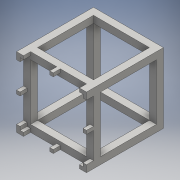
# Autodesk Inventor part: Kens_cube_of_fun_design_withpegs_spencermical
Saved by Autodesk Inventor 2016 (Build 200138000, 138)
## iProperties
Created: 2016-02-27
Part Number: Kens_cube_of_fun_design_withpegs_spencermical
Material: Generic
Document SubType Name: Modeling
Designer: Spencer
Density: 1 g/cm^3
Appearance: Default
Author: Spencer
Autodesk Inventor part; units mm, degrees
ref_plane "YZ Plane" through (0, 0, 0) normal (1, 0, 0) x (0, 1, 0)
ref_plane "XZ Plane" through (0, 0, 0) normal (0, 1, 0) x (-1, 0, 0)
ref_plane "XY Plane" through (0, 0, 0) normal (0, 0, 1) x (1, 0, 0)
sketch "Sketch1" plane through (0, 0, 0) normal (0, 1, 0) x (-1, 0, 0)
  line L0 (50, -50) -> (-50, -50)
  line L1 (-50, -50) -> (-50, 50)
  line L2 (-50, 50) -> (50, 50)
  line L3 (50, 50) -> (50, -50)
  point P0 (0, 0)
  dimension "d0" = 100
  dimension "d1" = 100
  dimension "d2" = 50
  dimension "d3" = 50
  constraints: 8 end point, 2 parallel, 1 horizontal, 1 perpendicular
  measures "d0" distance of L0.start L0.end
  measures "d1" distance of L2.end L0.start
  measures "d2" horizontal distance of L0.end point (0, 0)
  measures "d3" distance from line of L2 point (0, 0)
extrude "Extrusion1" add sketch "Sketch1" along normal blind 100
sketch "Sketch2" plane through (-50, 0, 50) normal (0, 0, 1) x (1, 0, 0)
  line L0 (10, 90) -> (90, 90)
  line L1 (90, 90) -> (90, 10)
  line L2 (90, 10) -> (10, 10)
  line L3 (10, 10) -> (10, 90)
  line L4 (100, 0) -> (0, 0) projected
  line L5 (100, 0) -> (100, 100) projected
  point P0 (50, 0)
  dimension "d6" = 80
  dimension "d7" = 10
  dimension "d8" = 80
  dimension "d9" = 10
  constraints: 8 end point, 2 parallel, 1 horizontal, 1 perpendicular
  measures "d6" distance of L2.end L0.start
  measures "d7" distance from line of L4 L2.end
  measures "d8" distance of L1.end L2.end
  measures "d9" distance from line of L5 L1.end
extrude "Extrusion2" cut sketch "Sketch2" against normal blind 100
sketch "Sketch3" plane through (50, 0, 50) normal (1, 0, 0) x (0, 0, -1)
  line L0 (10, 90) -> (90, 90)
  line L1 (90, 90) -> (90, 10)
  line L2 (90, 10) -> (10, 10)
  line L3 (10, 10) -> (10, 90)
  line L4 (0, 100) -> (100, 100) projected
  line L5 (100, 0) -> (100, 100) projected
  point P0 (50, 0)
  dimension "d12" = 80
  dimension "d13" = 10
  dimension "d14" = 80
  dimension "d15" = 10
  constraints: 8 end point, 2 parallel, 1 horizontal, 1 perpendicular
  measures "d12" distance of L2.end L0.start
  measures "d13" distance from line of L4 L0.start
  measures "d14" distance of L0.start L0.end
  measures "d15" distance from line of L5 L1.end
extrude "Extrusion3" cut sketch "Sketch3" against normal blind 100
sketch "Sketch4" plane through (0, 100, 0) normal (0, 1, 0) x (1, 0, 0)
  line L0 (-40, -50) -> (-40, -40) projected
  line L1 (50, 40) -> (40, 40) projected
  line L2 (-40, -40) -> (40, -40)
  line L3 (40, -40) -> (40, 40)
  line L4 (40, 40) -> (-40, 40)
  line L5 (-40, 40) -> (-40, -40)
  point P0 (0, 0)
  constraints: 8 end point, 2 parallel, 1 horizontal, 1 perpendicular
extrude "Extrusion4" cut sketch "Sketch4" against normal blind 100
sketch "Sketch9" plane through (0, 0, 0) normal (0, -1, 0) x (1, 0, 0)
  line L0 (50, 0.0049) -> (45, 0.0049)
  line L1 (45, 0.0049) -> (45, -2.4951)
  line L2 (45, -2.4951) -> (50, -2.4951)
  line L3 (50, -2.4951) -> (50, 0.0049)
  line L4 (40, 40) -> (40, -40) projected
  point P0 (0, 0)
  dimension "d40" = 5
  dimension "d41" = 5
  dimension "d42" = 2.5
  constraints: 8 end point, 2 parallel, 1 horizontal, 1 perpendicular
  measures "d40" distance from line of L4 L1.end
  measures "d41" distance of L1.end L2.end
  measures "d42" distance of L0.end L1.end
sketch "Sketch10" plane through (0, 0, 0) normal (0, -1, 0) x (1, 0, 0)
  line L0 (50, -40) -> (50, 40) projected
  line L1 (50, 0) -> (45, 0)
  line L2 (45, 0) -> (45, 2.5)
  line L3 (45, 2.5) -> (50, 2.5)
  line L4 (50, 2.5) -> (50, 0)
  line L5 (40, 40) -> (40, -40) projected
  point P0 (0, 0)
  dimension "d43" = 2.5
  dimension "d44" = 5
  constraints: 8 end point, 2 parallel, 1 horizontal, 1 midpoint, 1 perpendicular
  measures "d43" distance of L1.end L2.end
  measures "d44" distance from line of L5 L2.end
extrude "Extrusion9" add sketch "Sketch9" along normal blind 10
extrude "Extrusion10" add sketch "Sketch10" along normal blind 10
mirror "Mirror3" about plane through (0, 0, 0) normal (1, 0, 0) of "Extrusion9", "Extrusion10"
sketch "Sketch11" plane through (0, 0, 0) normal (0, -1, 0) x (1, 0, 0)
  line L0 (-40, -50) -> (40, -50) projected
  line L1 (0, -50) -> (-2.5, -50)
  line L2 (-2.5, -50) -> (-2.5, -45)
  line L3 (-2.5, -45) -> (0, -45)
  line L4 (0, -45) -> (0, -50)
  line L5 (40, -40) -> (-40, -40) projected
  point P0 (0, 0)
  dimension "d49" = 5
  dimension "d50" = 2.5
  constraints: 8 end point, 2 parallel, 1 horizontal, 1 midpoint, 1 perpendicular
  measures "d49" distance from line of L5 L2.end
  measures "d50" distance of L2.end L3.end
sketch "Sketch12" plane through (0, 0, 0) normal (0, -1, 0) x (1, 0, 0)
  line L0 (-40, -50) -> (40, -50) projected
  line L1 (0, -50) -> (2.5, -50)
  line L2 (2.5, -50) -> (2.5, -45)
  line L3 (2.5, -45) -> (0, -45)
  line L4 (0, -45) -> (0, -50)
  line L5 (40, -40) -> (-40, -40) projected
  point P0 (0, 0)
  dimension "d51" = 5
  dimension "d52" = 2.5
  constraints: 8 end point, 2 parallel, 1 horizontal, 1 midpoint, 1 perpendicular
  measures "d51" distance from line of L5 L2.end
  measures "d52" distance of L2.end L3.end
extrude "Extrusion11" add sketch "Sketch11" along normal blind 10
extrude "Extrusion12" add sketch "Sketch12" along normal blind 10
mirror "Mirror4" about plane through (0, 0, 0) normal (0, 0, 1) of "Extrusion11", "Extrusion12"
sketch "Sketch13" plane through (0, 0, 0) normal (0, -1, 0) x (1, 0, 0)
  line L0 (50, -40) -> (50, 40) projected
  line L1 (50, -50) -> (-50, -50) projected
  line L2 (50, -40) -> (45, -40)
  line L3 (45, -40) -> (45, -50)
  line L4 (45, -50) -> (50, -50)
  line L5 (50, -50) -> (50, -40)
  line L6 (40, 40) -> (40, -40) projected
  line L7 (45, -45) -> (40, -45)
  line L8 (40, -45) -> (40, -50)
  line L9 (40, -50) -> (45, -50)
  line L10 (45, -50) -> (45, -45)
  point P0 (0, 0)
  dimension "d57" = 5
  constraints: 16 end point, 4 parallel, 2 horizontal, 2 perpendicular, 1 midpoint, 1 point on line
  measures "d57" distance from line of L6 L2.end
extrude "Extrusion13" add sketch "Sketch13" along normal blind 10
mirror "Mirror5" about plane through (0, 0, 0) normal (0, 0, 1) of "Extrusion13"
mirror "Mirror6" about plane through (0, 0, 0) normal (1, 0, 0) of "Extrusion13"
mirror "Mirror7" about plane through (0, 0, 0) normal (0, 0, 1) of "Extrusion13", "Mirror6"
body "Solid1"
